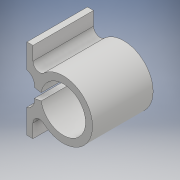
# Autodesk Inventor part: motor_holder
Saved by Autodesk Inventor 2017 (Build 210142000, 142)
## iProperties
Created: 2017-04-03
Part Number: motor_holder
Material: Generic
Document SubType Name: Modeling
Designer: Nick
Density: 1 g/cm^3
Appearance: Default
Author: Nick
Autodesk Inventor part; units mm, degrees
ref_plane "YZ Plane" through (0, 0, 0) normal (1, 0, 0) x (0, 1, 0)
ref_plane "XZ Plane" through (0, 0, 0) normal (0, 1, 0) x (-1, 0, 0)
ref_plane "XY Plane" through (0, 0, 0) normal (0, 0, 1) x (1, 0, 0)
sketch "Sketch1" plane through (0, 0, 0) normal (0, 1, 0) x (-1, 0, 0)
  arc A0 (10.9086, 1.7618) -> (10.9086, -1.7618) centre (0, 0) ccw
  arc A1 (14.3065, 2.361) -> (14.3065, -2.361) centre (0, 0) ccw
  line L0 (15, 13.2439) -> (15, 20)
  line L1 (15, 20) -> (18, 20)
  line L2 (18, 20) -> (18, 8)
  line L3 (15, -13.2439) -> (15, -20)
  line L4 (15, -20) -> (18, -20)
  line L5 (18, -20) -> (18, -8)
  arc A2 (9.6355, 10.8355) -> (15, 13.2439) centre (11.7771, 13.2439) ccw
  arc A3 (15, -13.2439) -> (9.6355, -10.8355) centre (11.7771, -13.2439) ccw
  line L6 (10.9086, -1.7618) -> (14.3065, -2.361)
  line L7 (10.9086, 1.7618) -> (14.3065, 2.361)
  line L8 (17.4762, 0) -> (-4.0395, 0) construction
  arc A4 (18, 8) -> (14.3065, 2.361) centre (19.2199, 3.1718) ccw
  arc A5 (14.3065, -2.361) -> (18, -8) centre (19.2199, -3.1718) ccw
  dimension "d0" = 22.1
  dimension "d1" = 29
  dimension "d2" = 12
  dimension "d3" = 12
  dimension "d4" = 3
  dimension "d5" = 3
  dimension "d8" = 15
  dimension "d10" = 10
  dimension "d11" = 10
  dimension "d12" = 3.5237
  dimension "d13" = 1.7618
  dimension "d14" = 20
  dimension "d15" = 20
  constraints: 18 end point, 14 point on circle, 6 centre point, 6 tangent, 4 perpendicular, 2 coincident, 2 equal radius, 1 collinear, 1 horizontal, 1 vertical
  measures "d0" diameter of A0
  measures "d1" diameter of A1
  measures "d2" distance of L1.end L2.end
  measures "d3" distance of L4.end L5.end
  measures "d4" distance of L0.end L1.end
  measures "d5" distance of L3.end L4.end
  measures "d8" distance from line of point (0, 0) L0
  measures "d10" angle of L6 L8
  measures "d11" angle of L7 L8
  measures "d12" distance of L7.start L6.start
  measures "d13" vertical distance of A0.centre L7.start
  measures "d14" vertical distance of point (0, 0) L3.end
  measures "d15" vertical distance of point (0, 0) L0.end
extrude "Extrusion1" add sketch "Sketch1" along normal blind 30
equation "\"d3\" = d2"
equation "\"d11\" = d10"
equation "\"d13\" = 0.5 * d12"
body "Solid1"
